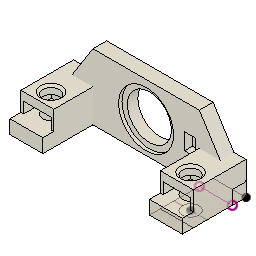
encoder-bracket (Autodesk Fusion 360 design; units mm, degrees)
Autodesk Fusion 360 part; units mm, degrees
sketch "Sketch1" plane through (0, 0, 0) normal (0, 0, 1) x (1, 0, 0)
  line L0 (-19.939, 0) -> (-19.939, 3.175)
  line L1 (-19.939, 3.175) -> (-12.319, 15.24)
  line L2 (-12.319, 15.24) -> (12.319, 15.24)
  line L3 (12.319, 15.24) -> (19.939, 3.175)
  line L4 (19.939, 3.175) -> (19.939, 0)
  line L5 (19.939, 0) -> (-19.939, 0)
  line L6 (0, 0) -> (0, 15.24) construction
  circle A0 centre (0, 7.3025) radius 5.08
  circle A1 centre (0, 7.3025) radius 6.35
  line L7 (8.89, 9.2075) -> (11.43, 9.2075)
  line L8 (11.43, 9.2075) -> (11.43, 5.3975)
  line L9 (11.43, 5.3975) -> (8.89, 5.3975)
  line L10 (8.89, 5.3975) -> (8.89, 9.2075)
  line L11 (10.16, 9.2075) -> (10.16, 5.3975) construction
  line L12 (0, 7.3025) -> (10.16, 7.3025) construction
  dimension "d1" = 39.878
  dimension "d2" = 3.175
  dimension "d3" = 7.62
  dimension "d4" = 15.24
  dimension "d5" = 10.16
  dimension "d6" = 7.3025
  dimension "d7" = 12.7
  dimension "d8" = 3.81
  dimension "d9" = 2.54
  dimension "d10" = 10.16
  measures "d4" distance of L2 L5
  measures "d5" diameter of A0
  measures "d6" distance of L6.start
  measures "d7" diameter of A1
extrude "Extrude1" add sketch "Sketch1" against normal blind 3.175 contours L0 L1 L2 L3 L4 L5 | A1 | L7 L8 L9 L10 makes body 1
extrude "Extrude2" cut sketch "Sketch1" against normal blind 0.762 contours A1 bodies 1
extrude "Extrude3" cut sketch "Sketch1" against normal blind 1.905 contours L7 L8 L9 L10 bodies 1
sketch "Sketch3" plane through (0, 0, 0) normal (0, 1, 0) x (1, 0, 0)
  line L0 (19.939, 3.175) -> (12.319, 3.175)
  line L1 (12.319, 3.175) -> (12.319, -9.017)
  line L2 (12.319, -9.017) -> (19.939, -9.017)
  line L3 (19.939, -9.017) -> (19.939, 3.175)
  line L4 (12.319, -5.842) -> (19.939, -5.842) construction
  circle A0 centre (16.129, -5.842) radius 1.905
  line L5 (12.319, 0) -> (19.939, 0)
  line L6 (12.319, -9.017) -> (19.939, -9.017)
  line L7 (19.939, -9.017) -> (19.939, -11.557)
  line L8 (19.939, -11.557) -> (12.319, -11.557)
  line L9 (12.319, -11.557) -> (12.319, -9.017)
  dimension "d17" = 12.192
  dimension "d18" = 7.62
  dimension "d19" = 3.81
  dimension "d21" = 5.842
  dimension "d31" = 2.54
  measures "d19" diameter of A0
  measures "d21" distance of L4 L5
extrude "Extrude4" add sketch "Sketch3" along normal blind 7.62 separate body contours L0 L1 L3 L5 | L1 L2 L3 L5 L6 makes body 2
extrude "Extrude6" add sketch "Sketch3" along normal blind 3.175 contours L2 L6 L7 L8 L9 bodies 2
sketch "Sketch4" plane through (0, 0, 9.017) normal (0, 0, 1) x (1, 0, 0)
  line L0 (19.939, 3.175) -> (19.939, 7.62)
  line L1 (19.939, 7.62) -> (12.319, 7.62)
  line L2 (12.319, 7.62) -> (12.319, 3.175)
  line L3 (12.954, 5.715) -> (19.304, 5.715)
  line L4 (19.304, 5.715) -> (19.304, 3.175)
  line L5 (19.304, 3.175) -> (12.954, 3.175)
  line L6 (12.954, 3.175) -> (12.954, 5.715)
  line L7 (16.129, 7.62) -> (16.129, 5.715) construction
  line L8 (12.319, 3.175) -> (19.939, 3.175)
  dimension "d24" = 6.35
  dimension "d25" = 2.54
extrude "Extrude5" cut sketch "Sketch4" against normal blind 6.35 contours L3 L4 L5 L6 L8 bodies 2
chamfer "Chamfer1" distance 0.508 angle 45 2 edges at (14.3529, 7.62, 5.1531) (14.3529, 0, 5.1531) on bodies 2
mirror "Mirror1" about plane through (0, 0, 0) normal (1, 0, 0) of "Extrude4", "Extrude6", "Extrude5", "Chamfer1" makes body 3
